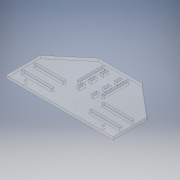
# Autodesk Inventor part: phone_holder_back
Saved by Autodesk Inventor 2019 (Build 230136000, 136)
## iProperties
Created: 2019-02-17
Part Number: phone_holder_back
Material: Acrylic, Clear
Document SubType Name: Modeling
Designer: suchanek
Density: 1.19 g/cm^3
Appearance: Transparent - Clear
Author: suchanek
Autodesk Inventor part; units mm, degrees
ref_plane "YZ Plane" through (0, 0, 0) normal (1, 0, 0) x (0, 1, 0)
ref_plane "XZ Plane" through (0, 0, 0) normal (0, 1, 0) x (-1, 0, 0)
ref_plane "XY Plane" through (0, 0, 0) normal (0, 0, 1) x (1, 0, 0)
sketch "Sketch2" plane through (0, 0, 0) normal (0, 1, 0) x (-1, 0, 0)
  line L0 (110, 62.5) -> (-110, 62.5)
  line L1 (-110, 62.5) -> (-110, -62.5)
  line L2 (-110, -62.5) -> (110, -62.5)
  line L3 (110, -62.5) -> (110, 62.5)
  line L4 (110, 62.5) -> (-110, -62.5) construction
  line L5 (-110, 62.5) -> (110, -62.5) construction
  line L6 (11.5, -50.5) -> (17.5, -50.5)
  line L7 (17.5, -50.5) -> (17.5, -38.5)
  line L8 (17.5, -38.5) -> (11.5, -38.5)
  line L9 (11.5, -38.5) -> (11.5, -50.5)
  line L10 (11.5, -26.5) -> (17.5, -26.5)
  line L11 (17.5, -26.5) -> (17.5, -14.5)
  line L12 (17.5, -14.5) -> (11.5, -14.5)
  line L13 (11.5, -14.5) -> (11.5, -26.5)
  line L14 (11.5, -2.5) -> (17.5, -2.5)
  line L15 (17.5, -2.5) -> (17.5, 9.5)
  line L16 (17.5, 9.5) -> (11.5, 9.5)
  line L17 (11.5, 9.5) -> (11.5, -2.5)
  line L18 (-17.5, -50.5) -> (-11.5, -50.5)
  line L19 (-11.5, -50.5) -> (-11.5, -38.5)
  line L20 (-11.5, -38.5) -> (-17.5, -38.5)
  line L21 (-17.5, -38.5) -> (-17.5, -50.5)
  line L22 (-17.5, -26.5) -> (-11.5, -26.5)
  line L23 (-11.5, -26.5) -> (-11.5, -14.5)
  line L24 (-11.5, -14.5) -> (-17.5, -14.5)
  line L25 (-17.5, -14.5) -> (-17.5, -26.5)
  line L26 (-17.5, -2.5) -> (-11.5, -2.5)
  line L27 (-11.5, -2.5) -> (-11.5, 9.5)
  line L28 (-11.5, 9.5) -> (-17.5, 9.5)
  line L29 (-17.5, 9.5) -> (-17.5, -2.5)
  line L30 (0, 0) -> (0, -18.9718)
  line L31 (25, -2.5) -> (25, -52.5) construction
  line L32 (22.4, -2.5) -> (22.4, -52.5)
  line L33 (27.6, -52.5) -> (27.6, -2.5)
  arc A0 (27.6, -2.5) -> (22.4, -2.5) centre (25, -2.5) ccw
  arc A1 (22.4, -52.5) -> (27.6, -52.5) centre (25, -52.5) ccw
  line L34 (100, 12.5) -> (40, 12.5) construction
  line L35 (100, 15.1) -> (40, 15.1)
  line L36 (40, 9.9) -> (100, 9.9)
  arc A2 (100, 9.9) -> (100, 15.1) centre (100, 12.5) ccw
  arc A3 (40, 15.1) -> (40, 9.9) centre (40, 12.5) ccw
  line L37 (100, 37.5) -> (40, 37.5) construction
  line L38 (100, 40.1) -> (40, 40.1)
  line L39 (40, 34.9) -> (100, 34.9)
  arc A4 (100, 34.9) -> (100, 40.1) centre (100, 37.5) ccw
  arc A5 (40, 40.1) -> (40, 34.9) centre (40, 37.5) ccw
  line L40 (-25, -2.5) -> (-25, -52.5) construction
  line L41 (-22.4, -2.5) -> (-22.4, -52.5)
  line L42 (-27.6, -52.5) -> (-27.6, -2.5)
  arc A6 (-22.4, -2.5) -> (-27.6, -2.5) centre (-25, -2.5) ccw
  arc A7 (-27.6, -52.5) -> (-22.4, -52.5) centre (-25, -52.5) ccw
  line L43 (-100, 12.5) -> (-40, 12.5) construction
  line L44 (-100, 15.1) -> (-40, 15.1)
  line L45 (-40, 9.9) -> (-100, 9.9)
  arc A8 (-100, 15.1) -> (-100, 9.9) centre (-100, 12.5) ccw
  arc A9 (-40, 9.9) -> (-40, 15.1) centre (-40, 12.5) ccw
  line L46 (-100, 37.5) -> (-40, 37.5) construction
  line L47 (-100, 40.1) -> (-40, 40.1)
  line L48 (-40, 34.9) -> (-100, 34.9)
  arc A10 (-100, 40.1) -> (-100, 34.9) centre (-100, 37.5) ccw
  arc A11 (-40, 34.9) -> (-40, 40.1) centre (-40, 37.5) ccw
  circle A12 centre (80, 52.5) radius 2.6
  circle A13 centre (-80, 52.5) radius 2.6
  line L49 (110, -7.5) -> (45, -62.5)
  line L50 (-45, -62.5) -> (-110, -7.5)
  point P0 (25, -27.5)
  point P1 (70, 12.5)
  point P2 (70, 37.5)
  point P3 (-25, -27.5)
  point P4 (-70, 12.5)
  point P5 (-70, 37.5)
  dimension "d52" = 220
  dimension "d53" = 125
  dimension "d54" = 12
  dimension "d55" = 6
  dimension "d58" = 24
  dimension "d61" = 29
  dimension "d65" = 12
  dimension "d66" = 5.2
  dimension "d68" = 100
  dimension "d69" = 115
  dimension "d70" = 40
  dimension "d71" = 65
  dimension "d72" = 15
  dimension "d73" = 25
  dimension "d75" = 15
  dimension "d76" = 5.2
  dimension "d79" = 30
  dimension "d80" = 10
  dimension "d81" = 20
  dimension "d82" = 20
  constraints: 114 end point, 24 point on circle, 23 symmetric about line, 14 centre point, 12 tangent, 8 parallel, 5 midpoint, 4 point on line, 3 horizontal, 3 perpendicular, 3 vertical, 2 equal radius, 2 vertical alignment, 1 horizontal alignment, 48 other
  measures "d52" distance of L2.end L1.end
  measures "d53" distance of L1.end L0.end
  measures "d54" distance of L8.end L6.start
  measures "d55" distance of L6.start L6.end
  measures "d58" distance of L6.start L10.start
  measures "d61" distance of L6.start L18.start
  measures "d65" distance between parallel lines of L2 L6
  measures "d66" diameter of A1
  measures "d68" distance from line of L30 L34.start
  measures "d69" distance from line of L0 L31.end
  measures "d70" distance from line of L30 L34.end
  measures "d71" distance from line of L0 L31.start
  measures "d72" horizontal distance of L31.start L34.end
  measures "d73" distance from line of L0 L37.end
  measures "d75" horizontal distance of L31.start L34.end
  measures "d76" diameter of A12
  measures "d79" distance from line of L3 A12.centre
  measures "d80" distance from line of L0 A12.centre
  measures "d81" distance from line of L49.end L31
  measures "d82" distance from line of L49.start L34
extrude "Extrusion2" add sketch "Sketch2" along normal blind 6 contours L3 L49 L2 L50 L1 L0
body "Solid2"
